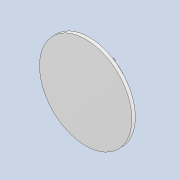
# Autodesk Inventor part: Lid_plain
Saved by Autodesk Inventor 2020.2 (Build 242310000, 310)
## iProperties
Created: 2021-08-27
Part Number: Lid_plain
Material: PC/ABS-Kunststoff
Document SubType Name: Modeling
Designer: johan
Density: 0.357273 g/cm^3
Appearance: Glatt - Weiß
Author: johan
Autodesk Inventor part; units mm, degrees
ref_plane "YZ Plane" through (0, 0, 0) normal (1, 0, 0) x (0, 1, 0)
ref_plane "XZ Plane" through (0, 0, 0) normal (0, 1, 0) x (-1, 0, 0)
ref_plane "XY Plane" through (0, 0, 0) normal (0, 0, 1) x (1, 0, 0)
sketch "Skizze1" plane through (0, 0, 0) normal (0, 0, 1) x (1, 0, 0)
  circle A0 centre (0, 0) radius 12.3
  arc A1 (13.4907, -0.4999) -> (13.4907, 0.4999) centre (13.5, 0) ccw
  arc A2 (-13.4907, -0.4999) -> (13.4907, -0.4999) centre (0, 0) ccw
  line L0 (0, -18.9) -> (0, 18.9) construction
  line L1 (-20.7866, 0) -> (20.7866, 0) construction
  arc A3 (7.1783, 11.4334) -> (6.3124, 11.9333) centre (6.75, 11.6913) ccw
  arc A4 (-6.3124, 11.9333) -> (-7.1783, 11.4334) centre (-6.75, 11.6913) ccw
  arc A5 (-13.4907, 0.4999) -> (-13.4907, -0.4999) centre (-13.5, 0) ccw
  arc A6 (-7.1783, -11.4334) -> (-6.3124, -11.9333) centre (-6.75, -11.6913) ccw
  arc A7 (6.3124, -11.9333) -> (7.1783, -11.4334) centre (6.75, -11.6913) ccw
  arc A8 (13.4907, 0.4999) -> (7.1783, 11.4334) centre (0, 0) ccw
  arc A9 (6.3124, 11.9333) -> (-6.3124, 11.9333) centre (0, 0) ccw
  arc A10 (-7.1783, 11.4334) -> (-13.4907, 0.4999) centre (0, 0) ccw
  point P0 (-13.4907, -0.4999)
  point P1 (-6.3124, -11.9333)
  dimension "d3" = 0
  dimension "d7" = 1
  dimension "d9" = 13.5
  dimension "d10" = 24.6
  dimension "d11" = 13.5
  dimension "d12" = 0
  dimension "d13" = 13.4907
  dimension "d14" = 13.4907
  dimension "d69" = 360
  constraints: 20 point on circle, 11 centre point, 25 other
  measures "d3" distance of point (0, 0) A0.centre
  measures "d7" diameter of A1
  measures "d9" radius of A2
  measures "d10" diameter of A0
  measures "d11" distance from line of A1.centre L0
  measures "d12" distance from line of A1.centre L1
  measures "d13" distance from line of A10.end L0
  measures "d14" distance from line of A2.start L0
extrude "Extrusion1" add sketch "Skizze1" along normal blind 1.8
sketch "Skizze2" plane through (0, 0, 1.8) normal (0, 0, 1) x (1, 0, 0)
  circle A0 centre (0, 0) radius 16
  dimension "d15" = 32
  constraints: 1 centre point, 1 coincident
  measures "d15" diameter of A0
extrude "Extrusion2" add sketch "Skizze2" along normal blind 1.2
